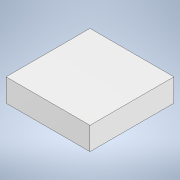
# Autodesk Inventor part: DCfan_small
Saved by Autodesk Inventor 2022 (Build 260153000, 153)
## iProperties
Created: 2022-06-14
Part Number: DCfan_small
Material: ABS プラスチック
Document SubType Name: Modeling
Designer: yuto6
Density: 1.06 g/cm^3
Appearance: 滑らか - 白
Author: yuto6
Autodesk Inventor part; units mm, degrees
ref_plane "YZ Plane" through (0, 0, 0) normal (1, 0, 0) x (0, 1, 0)
ref_plane "XZ Plane" through (0, 0, 0) normal (0, 1, 0) x (-1, 0, 0)
ref_plane "XY Plane" through (0, 0, 0) normal (0, 0, 1) x (1, 0, 0)
sketch "スケッチ1" plane through (0, 0, 0) normal (0, 1, 0) x (-1, 0, 0)
  line L0 (46, -46) -> (-46, -46)
  line L1 (-46, -46) -> (-46, 46)
  line L2 (-46, 46) -> (46, 46)
  line L3 (46, 46) -> (46, -46)
  line L4 (46, -46) -> (-46, 46) construction
  line L5 (-46, -46) -> (46, 46) construction
  point P0 (0, 0)
  dimension "d0" = 92
  dimension "d1" = 92
  constraints: 12 end point, 2 midpoint, 2 parallel, 1 horizontal, 1 perpendicular
  measures "d0" distance of L1.end L2.end
  measures "d1" distance of L2.end L0.start
extrude "押し出し1" add sketch "スケッチ1" along normal blind 25
equation "\"d1\" = d0"
